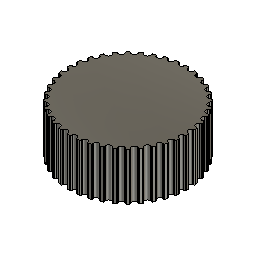
gear_40Z (Autodesk Fusion 360 design; units mm, degrees)
Autodesk Fusion 360 part; units mm, degrees
sketch "Sketch1" plane through (0, 0, 0) normal (0, 0, 1) x (1, 0, 0) in component "gt2 pulley"
  circle A0 centre (0, 0) radius 12.7324 construction
  circle A1 centre (0, 0) radius 11.7284 construction
  line L0 (0, 0) -> (0, 12.7324) construction
  line L1 (0, 0) -> (0.999, 12.6931) construction
  line L2 (0, 0) -> (1.4085, 12.6542) construction
  circle A2 centre (0, 0) radius 12.4784 construction
  arc A3 (0.3826, 12.3361) -> (0.4441, 12.0506) centre (1.3804, 12.4018) ccw
  circle A4 centre (0, 0) radius 12.3284 construction
  arc A5 (0.2357, 12.4762) -> (0, 12.4784) centre (0, 0) ccw
  arc A6 (0.3826, 12.3361) -> (0.2357, 12.4762) centre (0.2329, 12.3262) ccw
  arc A7 (0.4441, 12.0506) -> (0.9202, 11.6922) centre (0.9637, 12.2455) ccw
  arc A8 (0, 12.4784) -> (-0.2357, 12.4762) centre (0, 0) ccw
  arc A9 (-0.2357, 12.4762) -> (-0.3826, 12.3361) centre (-0.2329, 12.3262) ccw
  arc A10 (-0.4441, 12.0506) -> (-0.3826, 12.3361) centre (-1.3804, 12.4018) ccw
  arc A11 (-0.9202, 11.6922) -> (-0.4441, 12.0506) centre (-0.9637, 12.2455) ccw
  arc A12 (0.9202, 11.6922) -> (-0.9202, 11.6922) centre (0, 0) ccw
  point P0 (1.3804, 12.4018)
  point P1 (0, 12.4784)
  dimension "d18" = 25.4648
  dimension "d19" = 4.5
  dimension "d22" = 1.004
  dimension "d24" = 0.75
  dimension "d26" = 1
  dimension "d27" = 0.15
  dimension "d28" = 0.15
  dimension "d47" = 0.555
  dimension "d52" = 3.812
  constraint coincident A0.centre A1.centre
  constraint coincident A0 L0.end
  constraint vertical L0
  constraint coincident A0 L1.end
  constraint coincident A0 L2.end
  constraint concentric A1 A2
  constraint coincident A1 A7.end
  constraint coincident L1 A7.end
  constraint coincident A2 P0
  constraint coincident L2 P0
  constraint coincident P0 A3.centre
  constraint coincident A2 P1
  constraint coincident L0 P1
  constraint concentric A2 A4
  constraint coincident P1 A5.end
  constraint coincident A4 A6.centre
  constraint coincident A3.start A6.start
  constraint tangent A3 A6
  constraint tangent A3 A7
  constraint symmetric L0 A7.end A11.start
  constraint symmetric L0 A3.start A9.end
  constraint symmetric L0 A3.end A10.start
  constraint symmetric L0 A3 A10
  constraint symmetric L0 A5.start A8.end
  constraint symmetric L0 P1 A5.end
  constraint symmetric L0 A5 A8
  constraint symmetric L0 A6 A9
  constraint symmetric L0 A7 A11
  constraint coincident A1 A11.start
  constraint tangent A1 A7
  constraint coincident L1 A7.centre
  measures "d18" diameter of A0
  measures "d19" angle of L0 L1
  measures "d22" distance of A0 A1
  measures "d24" distance of A1 A2
  measures "d26" radius of A3
  measures "d27" distance of A2 A4
  measures "d28" radius of A6
  measures "d47" radius of A7
extrude "Extrude1" add sketch "Sketch1" along normal blind 7 makes body 1
pattern_circular "C-Pattern1" count 40 over 360 about axis through (0, 0, 1.75) along (0, 0, 1) of bodies 1 makes body 2 at (-1.1241, 11.6744, 2.3333) makes body 3 at (-4.2985, 10.9123, 4.6667) makes body 4 at (-5.4156, 10.4032, 4.6667) makes body 5 at (-7.4602, 9.0499, 4.6667) makes body 6 at (-7.7715, 8.784, 2.3333) makes body 7 at (-9.8916, 6.3017, 4.6667) makes body 8 at (-10.4961, 5.2332, 4.6667) makes body 9 at (-11.1856, 3.5268, 4.6667) makes body 10 at (-11.5996, 1.7336, 4.6667) makes body 11 at (-11.7279, -0.1023, 4.6667) makes body 12 at (-11.6744, -1.1241, 2.3333) makes body 13 at (-10.9123, -4.2985, 4.6667) makes body 14 at (-10.4032, -5.4156, 4.6667) makes body 15 at (-9.0499, -7.4602, 4.6667) makes body 16 at (-8.784, -7.7715, 2.3333) makes body 17 at (-6.3017, -9.8916, 4.6667) makes body 18 at (-5.2332, -10.4961, 4.6667) makes body 19 at (-4.2985, -10.9123, 2.3333) makes body 20 at (-1.7336, -11.5996, 4.6667) makes body 21 at (0.1023, -11.7279, 4.6667) makes body 22 at (1.1241, -11.6744, 2.3333) makes body 23 at (3.7215, -11.1223, 4.6667) makes body 24 at (4.6767, -10.7556, 2.3333) makes body 25 at (7.4602, -9.0499, 4.6667) makes body 26 at (7.7715, -8.784, 2.3333) makes body 27 at (9.5483, -6.8107, 4.6667) makes body 28 at (10.1055, -5.9526, 2.3333) makes body 29 at (11.1856, -3.5268, 4.6667) makes body 30 at (11.5996, -1.7336, 4.6667) makes body 31 at (11.7279, 0.1023, 4.6667) makes body 32 at (11.6744, 1.1241, 2.3333) makes body 33 at (11.1223, 3.7215, 4.6667) makes body 34 at (10.7556, 4.6767, 2.3333) makes body 35 at (9.0499, 7.4602, 4.6667) makes body 36 at (8.784, 7.7715, 2.3333) makes body 37 at (7.4602, 9.0499, 2.3333) makes body 38 at (4.6767, 10.7556, 4.6667) makes body 39 at (2.9366, 11.3548, 4.6667) makes body 40 at (2.5385, 11.4504, 2.3333)
sketch "Sketch2" plane through (0, 0, 7) normal (0, 0, 1) x (-1, 0, 0)
  arc A0 (-5.9413, -10.8178) -> (-5.874, -11.0094) centre (-5.8035, -10.877) ccw
  arc A1 (-5.874, -11.0094) -> (-5.4541, -11.2233) centre (0, 0) ccw
  arc A2 (-5.4541, -11.2233) -> (-5.2596, -11.1652) centre (-5.3885, -11.0884) ccw
  arc A3 (-5.0752, -10.9388) -> (-5.2596, -11.1652) centre (-4.4004, -11.6768) ccw
  arc A4 (-4.4883, -10.8356) -> (-5.0752, -10.9388) centre (-4.7007, -11.3484) ccw
  arc A5 (-6.1281, -10.0001) -> (-4.4883, -10.8356) centre (0, 0) ccw
  arc A6 (-5.8666, -10.5356) -> (-6.1281, -10.0001) centre (-6.4181, -10.4733) ccw
  arc A7 (-5.9413, -10.8178) -> (-5.8666, -10.5356) centre (-6.8602, -10.4234) ccw
  circle A8 centre (0, 0) radius 11.7284
  constraint concentric A1 A8
extrude "Extrude2" add sketch "Sketch2" against normal blind 7 contours A5 A8 bodies 1 2 3 4 5 6 7 8 9 10 11 12 13 14 15 16 17 18 19 20 21 22 23 24 25 26 27 28 29 30 31 32 33 34 35 36 37 38 39 40
extrude "Extrude3" add 1 faces at (2.0427, 3.3334, 7) along direction (0, 0, 1) blind 3 on bodies 1 bodies 1
extrude "Extrude4" [suppressed] in component "gt2 pulley"
pattern_circular "C-Pattern7" [suppressed] in component "gt2 pulley"
extrude "Extrude3'" [suppressed] in component "gt2 pulley"
pattern_circular "C-Pattern6" [suppressed] in component "gt2 pulley"
extrude "Extrude2'" [suppressed] in component "gt2 pulley"
pattern_circular "C-Pattern5" [suppressed] in component "gt2 pulley"
extrude "Extrude1'" [suppressed] in component "gt2 pulley"
pattern_circular "C-Pattern4" [suppressed] in component "gt2 pulley"
pattern_circular "C-Pattern3" [suppressed] in component "gt2 pulley"
pattern_circular "C-Pattern2" [suppressed] in component "gt2 pulley"
pattern_circular "C-Pattern1'" [suppressed] in component "gt2 pulley"
copy_body "Body->Comp1" [suppressed] in component "Component"
copy_body "Body->Comp2" [suppressed] in component "Component'"
copy_body "Body->Comp3" [suppressed] in component "Component''"
copy_body "Body->Comp4" [suppressed] in component "Component'''"
copy_body "Body->Comp5" [suppressed] in component "Component''''"
copy_body "Body->Comp6" [suppressed] in component "Component'''''"
copy_body "Body->Comp7" [suppressed] in component "Component''''''"
copy_body "Body->Comp8" [suppressed] in component "Component'''''''"
copy_body "Body->Comp9" [suppressed] in component "Component''''''''"
copy_body "Body->Comp10" [suppressed] in component "Component'''''''''"
copy_body "Body->Comp11" [suppressed] in component "Component''''''''''"
copy_body "Body->Comp12" [suppressed] in component "Component'''''''''''"
copy_body "Body->Comp13" [suppressed] in component "Component''''''''''''"
copy_body "Body->Comp14" [suppressed] in component "Component'''''''''''''"
copy_body "Body->Comp15" [suppressed] in component "Component''''''''''''''"
copy_body "Body->Comp16" [suppressed] in component "Component'''''''''''''''"
copy_body "Body->Comp17" [suppressed] in component "Component''''''''''''''''"
copy_body "Body->Comp18" [suppressed] in component "Component'''''''''''''''''"
copy_body "Body->Comp19" [suppressed] in component "Component''''''''''''''''''"
copy_body "Body->Comp20" [suppressed] in component "Component'''''''''''''''''''"
component "gt2 pulley" placed x (1, 0, 0) y (0, 1, 0) z (0, 0, 1) at (0, 0, 0)
equation "NumTeeth = 40" comment "min 20"
equation "ToothPitch = 2 mm"
equation "PullyDia = NumTeeth * ToothPitch / PI"
equation "ToothAng = ( ( 360 / NumTeeth ) * 1 deg )"
equation "TransOffsetAngle = ToothAng * 0.2"
equation "Sholulder_Radius = 0.15 mm"
equation "Root_Radius = 0.555 mm"
equation "TransRadius = 1 mm"
equation "ToolHeight = 0.75 mm"
equation "PLD = 0.254 mm"
equation "d18 = PullyDia"
equation "d19 = ToothAng / 2"
equation "d22 = PLD + ToolHeight"
equation "d24 = ToolHeight"
equation "d26 = TransRadius"
equation "d27 = Sholulder_Radius"
equation "d31 = NumTeeth"
equation "d33 = NumTeeth"
equation "d35 = NumTeeth"
equation "d37 = NumTeeth"
equation "d41 = NumTeeth"
equation "d45 = NumTeeth"
equation "d47 = Root_Radius"
equation "d50 = NumTeeth"
